Ladle Loop (Autodesk Fusion 360 design; units mm, degrees)
Autodesk Fusion 360 part; units mm, degrees
sketch "Sketch1" plane through (0, 0, 0) normal (0, 1, 0) x (1, 0, 0)
  circle A0 centre (0, 0) radius 8.1
  circle A1 centre (0, 0) radius 11.5
  dimension "d1" = 16.2
  dimension "d2" = 23
  constraint coincident A0.centre A1.centre
  constraint concentric A0 A1
  measures "d1" diameter of A0
  measures "d2" diameter of A1
extrude "Extrude1" add sketch "Sketch1" along normal blind 8 from surface at 2
extrude "Extrude2" add sketch "Sketch1" along normal blind 4 from surface at 10 contours A0 | A1
sketch "Sketch2" plane through (0, 0, 0) normal (0, 0, 1) x (1, 0, 0)
  ellipse E0 centre (0, 24) end of major axis (0, 31.5) minor radius 3.5
  line L0 (0, 16.5) -> (0, 31.5)
  line L1 (3.5, 24) -> (-3.5, 24)
  dimension "d8" = 15
  dimension "d9" = 7
  dimension "d10" = 24
  constraint coincident E0 L0.start
  constraint coincident E0 L0.end
  constraint coincident E0 L1.start
  constraint coincident E0 L1.end
  constraint vertical origin E0.centre
  measures "d8" distance of E0
  measures "d10" distance of origin E0.centre
sketch "Sketch3" plane through (0, 0, 0) normal (0, 0, 1) x (1, 0, 0)
  line L0 (6, 12) -> (-6, 12)
  line L1 (-6, 12) -> (-6, 35)
  line L2 (-6, 35) -> (6, 35)
  line L3 (6, 35) -> (6, 12)
  line L4 (6, 12) -> (-6, 35) construction
  line L5 (-6, 12) -> (6, 35) construction
  point P0 (0, 23.5)
  dimension "d11" = 12
  dimension "d12" = 23
  dimension "d13" = 12
  constraint perpendicular L0 L1
  constraint parallel L0 L2
  constraint parallel L1 L3
  constraint horizontal L0
  constraint coincident L4 P0
  constraint coincident L5 P0
  constraint vertical origin P0
  measures "d11" distance of L1.end L2.end
  measures "d12" distance of L0.end L1.end
  measures "d13" distance of L0 origin
extrude "Extrude3" add sketch "Sketch3" along normal mid plane 8
extrude "Extrude4" cut sketch "Sketch2" along normal mid plane 20
fillet "Fillet1" radius 2 8 edges at (6, 24.5, 4) (6, 24.5, -4) (0, 35, 4) (0, 35, -4) (6, 35, 0) (-6, 35, 0) (-6, 24.5, 4) (-6, 24.5, -4)
ref_plane "WorkPlane1" through (0, 10, 0) normal (0, -1, 0) x (-1, 0, 0)
